# Autodesk Inventor part: Roller Chain
Saved by Autodesk Inventor 2016 (Build 200138000, 138)
## iProperties
Created: 2017-01-14
Part Number: Roller Chain
Material: Generic
Document SubType Name: Modeling
Designer: katzchristy
Density: 1 g/cm^3
Appearance: Clear - Blue
CustomPartVersion: 1
Author: katzchristy
Autodesk Inventor part; units mm, degrees
ref_plane "Work Plane2" through (0, 0, 0) normal (-1, 0, 0) x (0, 0, 1)
ref_plane "Work Plane3" through (438.15, -76.2, 0) normal (-0.9048411, 0.4257495, 0) x (0, 0, 1)
sketch "Path" plane through (0, 0, 0) normal (0, 0, 1) x (1, 0, 0)
  arc A0 (19.6535, 74.3417) -> (-6.5993, -76.612) centre (0, 0) ccw
  arc A1 (434.839, -114.6373) -> (448.0104, -38.9017) centre (438.15, -76.2) ccw
  line L0 (434.839, -114.6373) -> (-6.5993, -76.612)
  line L1 (19.6535, 74.3417) -> (448.0104, -38.9017)
  dimension "d31" = 9.91
  constraints: 4 end point, 4 point on circle, 2 centre point
ref_plane "Section Plane" through (-6.5993, -76.612, 0) normal (0.9963105, -0.0858217, 0) x (0, 0, 1)
sketch "Section Sketch" plane through (-6.5993, -76.612, 0) normal (0.9963105, -0.0858217, 0) x (0, 0, 1)
  line L0 (-5.1, -1.83) -> (5.1, -1.83)
  line L1 (5.1, -1.83) -> (5.1, 1.83)
  line L2 (5.1, 1.83) -> (-5.1, 1.83)
  line L3 (-5.1, 1.83) -> (-5.1, -1.83)
  line L4 (-1.65, -3.875) -> (1.65, -3.875)
  line L5 (1.65, -3.875) -> (1.65, 3.875)
  line L6 (1.65, 3.875) -> (-1.65, 3.875)
  line L7 (-1.65, 3.875) -> (-1.65, -3.875)
  line L8 (-1.65, 0) -> (1.65, 0) construction
  line L9 (-3.65, -4.955) -> (-1.65, -4.955)
  line L10 (-1.65, -4.955) -> (-1.65, 4.955)
  line L11 (-1.65, 4.955) -> (-3.65, 4.955)
  line L12 (-3.65, 4.955) -> (-3.65, -4.955)
  line L13 (1.65, -4.955) -> (3.65, -4.955)
  line L14 (3.65, -4.955) -> (3.65, 4.955)
  line L15 (3.65, 4.955) -> (1.65, 4.955)
  line L16 (1.65, 4.955) -> (1.65, -4.955)
  line L17 (-5.1, 0) -> (5.1, 0) construction
  point P0 (0, 0)
  point P1 (0, 0)
  dimension "d21" = 3.66
  dimension "d22" = 7.75
  dimension "d23" = 3.3
  dimension "d24" = 2
  dimension "d31" = 9.91
  dimension "d32" = 10.2
  constraints: 36 end point, 8 midpoint, 8 parallel, 4 horizontal, 4 perpendicular, 3 collinear, 1 coincident, 1 other
  measures "d21" distance between parallel lines of L2 L0
  measures "d22" distance between parallel lines of L6 L4
  measures "d23" distance between parallel lines of L5 L7
  measures "d24" distance between parallel lines of L12 L10
  measures "d31" distance between parallel lines of L11 L9
  measures "d32" distance between parallel lines of L1 L3
sweep "Solid" add profiles "Section Sketch" path "Path"
pattern_of_one "Strand Pattern"
equation "\"d21\" = da_d2"
equation "\"d22\" = da_d1"
equation "\"d23\" = da_b1"
equation "\"d24\" = da_t1 + da_t2"
equation "\"d30\" = da_pt"
equation "\"da_p\" = 12.7"
equation "\"da_b1\" = 3.3"
equation "\"da_h2\" = 9.91"
equation "\"da_h3\" = 9.91"
equation "\"da_d1\" = 7.75"
equation "\"da_d2\" = 3.66"
equation "\"da_pt\" = 13.92"
equation "\"da_b\" = 10.2"
equation "\"da_t1\" = 1"
equation "\"da_t2\" = 1"
body "Solid1"
